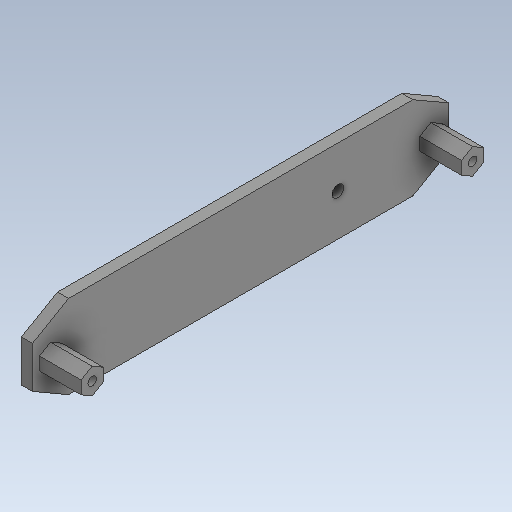
# Autodesk Inventor part: HexWheelGuard
Saved by Autodesk Inventor 2020 (Build 240168000, 168)
## iProperties
Created: 2023-12-19
Part Number: HexWheelGuard
Material: H TPU
Document SubType Name: Modeling
Designer: smz3rm
Density: 0.941117 g/cm^3
Appearance: Generic(1)
Mass: 17.2363 g
Surface Area: 118.102 cm^2
Volume: 18.3147 cm^3
Author: smz3rm
Autodesk Inventor part; units mm, degrees
ref_plane "YZ Plane" through (0, 0, 0) normal (1, 0, 0) x (0, 1, 0)
ref_plane "XZ Plane" through (0, 0, 0) normal (0, 1, 0) x (-1, 0, 0)
sketch "Sketch1" plane through (0, 0, 0) normal (1, 0, 0) x (0, 1, 0)
  line L0 (-15, 75) -> (15, 75)
  line L1 (15, 75) -> (15, -75)
  line L2 (15, -75) -> (-15, -75)
  line L3 (-15, -75) -> (-15, 75)
  line L4 (-15, 75) -> (15, -75) construction
  line L5 (15, 75) -> (-15, -75) construction
  line L6 (15, 64.89637) -> (15, 43.985813)
  line L7 (-15, 43.985813) -> (-15, 64.193072)
  line L8 (-21, 0) -> (21, 0)
  line L9 (0, -105) -> (0, 105)
  line L10 (-15, -62.009619) -> (-7.5, -49.019238)
  line L11 (-7.5, -49.019238) -> (7.5, -49.019238)
  line L12 (7.5, -49.019238) -> (15, -62.009619)
  line L13 (15, -62.009619) -> (7.5, -75)
  line L14 (7.5, -75) -> (-7.5, -75)
  line L15 (-7.5, -75) -> (-15, -62.009619)
  line L16 (15, 62.009619) -> (7.5, 75)
  line L17 (-7.5, 75) -> (-15, 62.009619)
  point P0 (0, 0)
  point P1 (0, -62.009619)
  point P2 (-7.5, -75)
  point P3 (7.5, -75)
  point P4 (15, -62.009619)
  point P5 (15, 62.009619)
  point P6 (7.5, 75)
  point P7 (-7.5, 75)
  point P8 (-15, 62.009619)
  dimension "d0" = 30
  dimension "d1" = 150
  constraints: 32 end point, 4 symmetric about line, 3 collinear, 2 midpoint, 2 parallel, 2 point on line, 1 horizontal, 1 perpendicular, 13 other
  measures "d0" distance of L1.end L2.end
  measures "d1" distance of L0.end L1.end
extrude "Extrusion1" add sketch "Sketch1" along normal blind 4 contours L0 L9 L8 L3 L17 | L0 L16 L1 L8 L9 | L9 L11 L10 L3 L8 | L8 L1 L12 L11 L9 | L11 L12 L13 L2 L9 | L9 L2 L15 L10 L11
sketch "Sketch2" plane through (4, 0, 0) normal (1, 0, 0) x (0, 0, -1)
  line L0 (62.009619, 15) -> (-62.009619, 15)
  line L1 (62.009619, 15) -> (-62.009619, 15)
  line L2 (-62.009619, -15) -> (62.009619, -15)
  line L3 (-105, 0) -> (105, 0)
  line L4 (0, -21) -> (0, 21)
  line L5 (-68.504809, 4.618802) -> (-64.504809, 2.309401)
  line L6 (-64.504809, 2.309401) -> (-64.504809, -2.309401)
  line L7 (-64.504809, -2.309401) -> (-68.504809, -4.618802)
  line L8 (-68.504809, -4.618802) -> (-72.504809, -2.309401)
  line L9 (-72.504809, -2.309401) -> (-72.504809, 2.309401)
  line L10 (-72.504809, 2.309401) -> (-68.504809, 4.618802)
  line L11 (68.504809, 4.618802) -> (64.504809, 2.309401)
  line L12 (64.504809, 2.309401) -> (64.504809, -2.309401)
  line L13 (64.504809, -2.309401) -> (68.504809, -4.618802)
  line L14 (68.504809, -4.618802) -> (72.504809, -2.309401)
  line L15 (72.504809, -2.309401) -> (72.504809, 2.309401)
  line L16 (72.504809, 2.309401) -> (68.504809, 4.618802)
  line L17 (-75, 7.5) -> (-75, -7.5)
  line L18 (-62.009619, -15) -> (62.009619, -15)
  line L19 (-62.009619, 15) -> (-62.009619, -15)
  line L20 (-75, 7.5) -> (-75, -7.5)
  line L21 (-75, 0) -> (-62.009619, 0)
  point P0 (0, 0)
  point P1 (68.504809, 0)
  point P2 (-68.504809, 0)
  dimension "d8" = 8
  constraints: 30 end point, 7 symmetric about line, 3 midpoint, 2 vertical, 1 point on line, 13 other
  measures "d8" distance between parallel lines of L6 L9
sketch "Sketch2 outline for Extrusion3" plane through (4, 0, 0) normal (1, 0, 0) x (0, 0, -1)
  line L0 (68.504809, -4.618802) -> (72.504809, -2.309401)
  line L1 (64.504809, -2.309401) -> (68.504809, -4.618802)
  line L2 (64.504809, 2.309401) -> (64.504809, -2.309401)
  line L3 (68.504809, 4.618802) -> (64.504809, 2.309401)
  line L4 (72.504809, 2.309401) -> (68.504809, 4.618802)
  line L5 (72.504809, -2.309401) -> (72.504809, 2.309401)
  line L6 (-64.504809, 2.309401) -> (-68.504809, 4.618802)
  line L7 (-64.504809, -2.309401) -> (-64.504809, 2.309401)
  line L8 (-68.504809, -4.618802) -> (-64.504809, -2.309401)
  line L9 (-72.504809, -2.309401) -> (-68.504809, -4.618802)
  line L10 (-72.504809, 2.309401) -> (-72.504809, -2.309401)
  line L11 (-68.504809, 4.618802) -> (-72.504809, 2.309401)
extrude "Extrusion3" add sketch "Sketch2 outline for Extrusion3" along normal blind 15
sketch "Sketch3" plane through (19, 0, 0) normal (1, 0, 0) x (0, 0, -1)
  line L0 (-64.504809, 2.309401) -> (-68.504809, 4.618802)
  line L1 (-68.504809, -4.618802) -> (-64.504809, -2.309401)
  line L2 (-64.504809, -2.309401) -> (-64.504809, 2.309401)
  line L3 (-64.504809, -2.309401) -> (-68.504809, -4.618802)
  circle A0 centre (-68.504809, 0) radius 1.55
  line L4 (0, -21) -> (0, 21)
  circle A1 centre (68.504809, 0) radius 1.55
  line L5 (-68.504809, 4.618802) -> (-68.504809, -4.618802)
  point P0 (0, 0)
  dimension "d12" = 3.1
  constraints: 2 centre point, 2 end point, 1 coincident, 1 midpoint, 1 symmetric about line, 1 vertical, 1 other
  measures "d12" diameter of A0
extrude "Extrusion4" cut sketch "Sketch3" against normal through all contours L5 A0 | A0 L5 | A1
ref_plane "Work Plane1" through (9, 0, 0) normal (1, 0, 0) x (0, 0, -1)
sketch "Sketch4" plane through (9, 0, 0) normal (-1, 0, 0) x (0, 0, 1)
  circle A0 centre (-68.504809, 0) radius 1.55
  circle A1 centre (68.504809, 0) radius 1.55
  circle A2 centre (-68.504809, 0) radius 3.05
  circle A3 centre (68.504809, 0) radius 3.05
  point P0 (0, 0)
  dimension "d15" = 6.1
  constraints: 2 centre point, 2 coincident, 1 equal radius
  measures "d15" diameter of A2
sketch "Sketch4 outline for Extrusion5" plane through (9, 0, 0) normal (-1, 0, 0) x (0, 0, 1)
  circle A0 centre (68.504809, 0) radius 3.05
  circle A1 centre (-68.504809, 0) radius 3.05
extrude "Extrusion5" cut sketch "Sketch4 outline for Extrusion5" against normal blind 2.2 draft -32.5
sketch "Sketch5" plane through (0, 0, 0) normal (-1, 0, 0) x (0, 0, 1)
  circle A0 centre (-68.504809, 0) radius 3.05
  circle A1 centre (68.504809, 0) radius 3.05
  point P0 (0, 0)
extrude "Extrusion6" cut sketch "Sketch5" against normal up to surface (9 mm away)
sketch "Sketch8" plane through (0, 0, 0) normal (-1, 0, 0) x (0, 0, 1)
  circle A0 centre (-35, 0) radius 2.1
  line L0 (-75, -7.5) -> (-75, 7.5) projected
  line L1 (0, -21) -> (0, 21) projected
  line L2 (75, 7.5) -> (75, -7.5) projected
  line L3 (-105, 0) -> (105, 0) projected
  point P0 (0, 0)
  dimension "d26" = 40
  dimension "d27" = 4.2
  constraints: 1 centre point, 1 point on line
  measures "d26" distance from line of L0 A0.centre
  measures "d27" diameter of A0
extrude "Extrusion7" cut sketch "Sketch8" against normal through all
equation "\"d0\" = BodyHeight"
equation "\"d1\" = BodyLength"
equation "\"d2\" = SideThickness"
equation "\"d8\" = M3ScrewInsertBrim"
equation "\"d9\" = WheeGuardlSlotWidth"
equation "\"d12\" = M3ScrewDia"
equation "\"d15\" = M3ScrewHeadDia"
equation "\"d16\" = M3ScrewHeadDepth"
equation "\"d17\" = M3ScrewHeadTaper"
equation "\"d26\" = DriveMotorOffset"
equation "\"d27\" = DriveMotorHoleDia"
equation "\"BodyHeight\" = 30"
equation "\"BodyLength\" = 150"
equation "\"SideThickness\" = 4"
equation "\"M3ScrewInsertBrim\" = 8"
equation "\"WheeGuardlSlotWidth\" = 15"
equation "\"M3ScrewDia\" = 3.1"
equation "\"M3ScrewHeadDia\" = 6.1"
equation "\"M3ScrewHeadDepth\" = 2.2"
equation "\"M3ScrewHeadTaper\" = -32.5deg"
equation "\"DriveMotorOffset\" = 40"
equation "\"DriveMotorHoleDia\" = 4.2"
body "Solid1"
